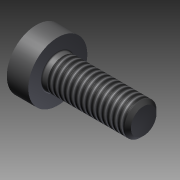
# Autodesk Inventor part: CBS3-8
Saved by Autodesk Inventor 2011 SP1 (Build 150282100, 282)
## iProperties
Created: 2016-04-08
Part Number: CBS3-8
Catalog Web Link: www.cadenas.de
Description: CBS, CBSST-Hexagon Socket Low Head Cap Screws
Vendor: MISUMI
Document SubType Name: Modeling
Designer: psAdmin
Manufacturer: MISUMI
Mass: 0.0980959 g
Surface Area: 1.65852 cm^2
Volume: 0.0980959 cm^3
Density: 1 g/cm^3
Category: PARTsolutions
Company: MISUMI
Title: CBS3-8
Author: Cadenas PARTsolutions
Comments: Hexagon Socket Low Head Cap Screws
PSOL_IDENT_0: {$CADENAS_DATA\23d-libs\misumi\metric\27_screws_nuts\cbsst.prj},163 {VTYP=3D},{NB=CBS3-8},{LINA=CBS3
PSOL_IDENT_1: -8},{NN=CBS, CBSST},{DATE=29.07.2015 04:50:04},{GEOMDATE=04.11.2010 00:00:00},{VERSION=},{LINEID=60}
PSOL_IDENT_2: ,{LINESUBID=-1},{WBVAR=MAT,L}  {NB=CBS3-8},{LINA=CBS3-8},{KT=DUMMY},{PN=CBS3-8},{MAT=},{MATA=  '','1
PSOL_IDENT_3: 045 Carbon Steel','ST','302HQ Stainless Steel'  },{HARD=22~32HRC},{ST=Black Oxide},{SC=8.8},{M=3},{L=
PSOL_IDENT_4: 8},{LL=Full Thread},{L1=40},{TYPE=CBS},{M1=3.000},{L0=6,8,10,12,16,20},{MP=3x0.5},{P=0.5},{A=5.5},{E=
PSOL_IDENT_5: 2.0},{B=2.0},{TT=1.5},{RR=0.1 or More},{RR1=0.10}
NN: CBS, CBSST
NT: Hexagon Socket Low Head Cap Screws
NB: CBS3-8
NBSYN: $PN.
LINA: CBS3-8
PN: CBS3-8
MAT: 1045 Carbon Steel
HARD: 22~32HRC
ST: Black Oxide
SC: 8.8
M: 3
L: 8
LL: Full Thread
MP: 3x0.5
A: 5.5
E: 2.0
B: 2.0
TT: 1.5
RR: 0.1 or More
SUPPLIER: MISUMI
ARTICLENO: CBS3-8
BOMINFO: CBS3-8
CREATOR: CADENAS GmbH
Autodesk Inventor part; units mm, degrees
sketch "Sketch_1" plane through (0, 0, 0) normal (0, 0, 1) x (1, 0, 0)
  line L0 (8, 0) -> (-2, 0)
  line L1 (-2, 0) -> (-2, 2.75)
  line L2 (-2, 2.75) -> (0, 2.75)
  line L3 (0, 2.75) -> (0, 1.6)
  arc A0 (0, 1.6) -> (0.1, 1.5) centre (0.1, 1.6) ccw
  line L4 (0.1, 1.5) -> (7.6935, 1.5)
  line L5 (7.6935, 1.5) -> (8, 1.1935)
  line L6 (8, 1.1935) -> (8, 0)
  line L7 (8, 0) -> (-2, 0)
  constraints: 16 end point, 2 point on circle, 1 centre point
revolve "Revolution1" add sketch "Sketch_1" angle 360 about axis through (8, 0, 0) along (1, 0, 0)
thread "Thread1" size "M3x0.5" class "6g" standard "ISO Metric profile" length 7.1935
sketch "Sketch2" plane through (-2, 0, 0) normal (-1, 0, 0) x (0, 0, 1)
  point P0 (0, 0)
hole "Hole1" at (-2, 0, 0) direction (1, 0, 0) diameter 2 depth 1.5 tip angle 140
sketch "Sketch_3" plane through (-2, 0, 0) normal (1, 0, 0) x (0, 0, -1)
  line L0 (-1, 0.5774) -> (-1, -0.5774)
  line L1 (-1, -0.5774) -> (0, -1.1547)
  line L2 (0, -1.1547) -> (1, -0.5774)
  line L3 (1, -0.5774) -> (1, 0.5774)
  line L4 (1, 0.5774) -> (0, 1.1547)
  line L5 (0, 1.1547) -> (-1, 0.5774)
  constraints: 12 end point
extrude "Extrusion1" cut sketch "Sketch_3" along normal blind 1.5
ref_plane "bolt_XY" through (0, 0, 0) normal (1, 0, 0) x (0, 0, -1)
ref_plane "bolt_YZ" through (0, 0, 0) normal (0, 0, -1) x (0, 1, 0)
ref_plane "bolt_ZX" through (0, 0, 0) normal (0, 1, 0) x (1, 0, 0)
ref_plane "bolt_to_nut_XY" through (8, 0, 0) normal (1, 0, 0) x (0, 0, -1)
ref_plane "bolt_to_nut_YZ" through (8, 0, 0) normal (0, 0, -1) x (0, 1, 0)
ref_plane "bolt_to_nut_ZX" through (8, 0, 0) normal (0, 1, 0) x (1, 0, 0)
body "Solid1"
